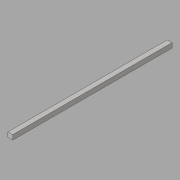
# Autodesk Inventor part: c1e
Saved by Autodesk Inventor 2016 (Build 200138000, 138)
## iProperties
Created: 2015-10-11
Part Number: c1e
Material: Generic
Document SubType Name: Modeling
Designer: daniel
Density: 1 g/cm^3
Appearance: Default
Author: daniel
Autodesk Inventor part; units mm, degrees
ref_plane "YZ Plane" through (0, 0, 0) normal (1, 0, 0) x (0, 1, 0)
ref_plane "XZ Plane" through (0, 0, 0) normal (0, 1, 0) x (-1, 0, 0)
ref_plane "XY Plane" through (0, 0, 0) normal (0, 0, 1) x (1, 0, 0)
derived "base.ipt"
sketch "sketch_projected_dwg" plane through (0, 0, 0) normal (0, 0, 1) x (1, 0, 0)
  line L0 (2002.0921, -140.1606) -> (2002.0921, -170.1606)
  line L1 (2002.0921, -170.1606) -> (2026.0921, -170.1606)
  line L2 (2026.0921, -170.1606) -> (2026.0921, -140.1606)
  line L3 (2026.0921, -140.1606) -> (2029.0921, -140.1606)
  line L4 (2029.0921, -140.1606) -> (2029.0921, -173.1606)
  line L5 (2029.0921, -173.1606) -> (2049.0921, -173.1606)
  line L6 (2049.0921, -173.1606) -> (2049.0921, -170.1606)
  line L7 (2049.0921, -170.1606) -> (2064.0921, -170.1606)
  line L8 (2064.0921, -170.1606) -> (2064.0921, -110.1606)
  line L9 (2064.0921, -110.1606) -> (2049.0921, -110.1606)
  line L10 (2049.0921, -110.1606) -> (2049.0921, -107.1606)
  line L11 (2049.0921, -107.1606) -> (2029.0921, -107.1606)
  line L12 (2029.0921, -107.1606) -> (2029.0921, -110.1606)
  line L13 (2029.0921, -110.1606) -> (1999.0921, -110.1606)
  line L14 (1999.0921, -110.1606) -> (1999.0921, -107.1606)
  line L15 (1999.0921, -107.1606) -> (1979.0921, -107.1606)
  line L16 (1979.0921, -107.1606) -> (1979.0921, -110.1606)
  line L17 (1979.0921, -110.1606) -> (1964.0921, -110.1606)
  line L18 (1964.0921, -110.1606) -> (1964.0921, -170.1606)
  line L19 (1964.0921, -170.1606) -> (1979.0921, -170.1606)
  line L20 (1979.0921, -170.1606) -> (1979.0921, -173.1606)
  line L21 (1979.0921, -173.1606) -> (1999.0921, -173.1606)
  line L22 (1999.0921, -173.1606) -> (1999.0921, -140.1606)
  line L23 (1999.0921, -140.1606) -> (2002.0921, -140.1606)
  line L24 (2002.0921, -228.8911) -> (2002.0921, -258.8911)
  line L25 (2002.0921, -258.8911) -> (1999.0921, -258.8911)
  line L26 (1999.0921, -258.8911) -> (1999.0921, -228.8911)
  line L27 (1999.0921, -228.8911) -> (1971.0921, -228.8911)
  line L28 (1971.0921, -228.8911) -> (1971.0921, -288.8911)
  line L29 (1971.0921, -288.8911) -> (2057.0921, -288.8911)
  line L30 (2057.0921, -288.8911) -> (2057.0921, -228.8911)
  line L31 (2057.0921, -228.8911) -> (2029.0921, -228.8911)
  line L32 (2029.0921, -228.8911) -> (2029.0921, -258.8911)
  line L33 (2029.0921, -258.8911) -> (2026.0921, -258.8911)
  line L34 (2026.0921, -258.8911) -> (2026.0921, -228.8911)
  line L35 (2026.0921, -228.8911) -> (2002.0921, -228.8911)
  circle A0 centre (2044.0921, -265.8911) radius 6
  circle A1 centre (2014.0921, -265.8911) radius 4.7571
  circle A2 centre (1984.0921, -265.8911) radius 6
  line L36 (2368.3683, 1.7867) -> (2368.3683, -98.2133)
  line L37 (2472.3683, 1.7867) -> (2472.3683, -98.2133)
  line L38 (2377.3683, -263.5692) -> (2377.3683, -363.5692)
  line L39 (2463.3683, -263.5692) -> (2463.3683, -363.5692)
  line L40 (2317.3683, -263.5692) -> (2377.3683, -263.5692)
  line L41 (2377.3683, -263.5692) -> (2420.3683, -263.5692)
  line L42 (2420.3683, -263.5692) -> (2463.3683, -263.5692)
  line L43 (2463.3683, -263.5692) -> (2523.3683, -263.5692)
  line L44 (2523.3683, -263.5692) -> (2523.3683, -333.5692)
  line L45 (2523.3683, -333.5692) -> (2493.3683, -363.5692)
  line L46 (2493.3683, -363.5692) -> (2347.3683, -363.5692)
  line L47 (2347.3683, -363.5692) -> (2317.3683, -333.5692)
  line L48 (2317.3683, -333.5692) -> (2317.3683, -263.5692)
  line L49 (2405.3683, -278.5692) -> (2408.3683, -278.5692)
  line L50 (2408.3683, -278.5692) -> (2408.3683, -298.5692)
  line L51 (2408.3683, -298.5692) -> (2405.3683, -298.5692)
  line L52 (2405.3683, -298.5692) -> (2405.3683, -278.5692)
  line L53 (2432.3683, -278.5692) -> (2435.3683, -278.5692)
  line L54 (2435.3683, -278.5692) -> (2435.3683, -298.5692)
  line L55 (2435.3683, -298.5692) -> (2432.3683, -298.5692)
  line L56 (2432.3683, -298.5692) -> (2432.3683, -278.5692)
  line L57 (2432.3683, -328.5692) -> (2435.3683, -328.5692)
  line L58 (2435.3683, -328.5692) -> (2435.3683, -348.5692)
  line L59 (2435.3683, -348.5692) -> (2432.3683, -348.5692)
  line L60 (2432.3683, -348.5692) -> (2432.3683, -328.5692)
  line L61 (2405.3683, -328.5692) -> (2408.3683, -328.5692)
  line L62 (2408.3683, -328.5692) -> (2408.3683, -348.5692)
  line L63 (2408.3683, -348.5692) -> (2405.3683, -348.5692)
  line L64 (2405.3683, -348.5692) -> (2405.3683, -328.5692)
  line L65 (2405.3683, -63.2133) -> (2408.3683, -63.2133)
  line L66 (2408.3683, -63.2133) -> (2408.3683, -83.2133)
  line L67 (2408.3683, -83.2133) -> (2405.3683, -83.2133)
  line L68 (2405.3683, -83.2133) -> (2405.3683, -63.2133)
  line L69 (2371.3683, -63.2133) -> (2374.3683, -63.2133)
  line L70 (2374.3683, -63.2133) -> (2374.3683, -83.2133)
  line L71 (2374.3683, -83.2133) -> (2371.3683, -83.2133)
  line L72 (2371.3683, -83.2133) -> (2371.3683, -63.2133)
  line L73 (2371.3683, -13.2133) -> (2374.3683, -13.2133)
  line L74 (2374.3683, -13.2133) -> (2374.3683, -33.2133)
  line L75 (2374.3683, -33.2133) -> (2371.3683, -33.2133)
  line L76 (2371.3683, -33.2133) -> (2371.3683, -13.2133)
  line L77 (2405.3683, -13.2133) -> (2408.3683, -13.2133)
  line L78 (2408.3683, -13.2133) -> (2408.3683, -33.2133)
  line L79 (2408.3683, -33.2133) -> (2405.3683, -33.2133)
  line L80 (2405.3683, -33.2133) -> (2405.3683, -13.2133)
  line L81 (2432.3683, -13.2133) -> (2435.3683, -13.2133)
  line L82 (2435.3683, -13.2133) -> (2435.3683, -33.2133)
  line L83 (2435.3683, -33.2133) -> (2432.3683, -33.2133)
  line L84 (2432.3683, -33.2133) -> (2432.3683, -13.2133)
  line L85 (2466.3683, -13.2133) -> (2469.3683, -13.2133)
  line L86 (2469.3683, -13.2133) -> (2469.3683, -33.2133)
  line L87 (2469.3683, -33.2133) -> (2466.3683, -33.2133)
  line L88 (2466.3683, -33.2133) -> (2466.3683, -13.2133)
  line L89 (2466.3683, -63.2133) -> (2469.3683, -63.2133)
  line L90 (2469.3683, -63.2133) -> (2469.3683, -83.2133)
  line L91 (2469.3683, -83.2133) -> (2466.3683, -83.2133)
  line L92 (2466.3683, -83.2133) -> (2466.3683, -63.2133)
  line L93 (2432.3683, -63.2133) -> (2435.3683, -63.2133)
  line L94 (2435.3683, -63.2133) -> (2435.3683, -83.2133)
  line L95 (2435.3683, -83.2133) -> (2432.3683, -83.2133)
  line L96 (2432.3683, -83.2133) -> (2432.3683, -63.2133)
  line L97 (2519.3683, -98.2133) -> (2469.3683, -98.2133)
  line L98 (2469.3683, 61.7867) -> (2519.3683, 61.7867)
  line L99 (2519.3683, 61.7867) -> (2519.3683, 1.7867)
  line L100 (2519.3683, 1.7867) -> (2595.3683, 1.7867)
  line L101 (2595.3683, 1.7867) -> (2595.3683, -13.2133)
  line L102 (2595.3683, -13.2133) -> (2598.3683, -13.2133)
  line L103 (2598.3683, -13.2133) -> (2598.3683, -33.2133)
  line L104 (2598.3683, -33.2133) -> (2595.3683, -33.2133)
  line L105 (2595.3683, -33.2133) -> (2595.3683, -48.2133)
  line L106 (2595.3683, -48.2133) -> (2595.3683, -63.2133)
  line L107 (2595.3683, -63.2133) -> (2598.3683, -63.2133)
  line L108 (2598.3683, -63.2133) -> (2598.3683, -83.2133)
  line L109 (2598.3683, -83.2133) -> (2595.3683, -83.2133)
  line L110 (2595.3683, -83.2133) -> (2595.3683, -98.2133)
  line L111 (2595.3683, -98.2133) -> (2519.3683, -98.2133)
  line L112 (2519.3683, -98.2133) -> (2519.3683, -158.2133)
  line L113 (2519.3683, -158.2133) -> (2394.6842, -158.2133)
  line L114 (2532.3683, 1.7867) -> (2532.3683, -98.2133)
  line L115 (2535.3683, 1.7867) -> (2535.3683, -98.2133)
  line L116 (2371.3683, -158.2133) -> (2371.3683, -98.2133)
  line L117 (2371.3683, -98.2133) -> (2469.3683, -98.2133)
  line L118 (2469.3683, -98.2133) -> (2469.3683, -158.2133)
  circle A3 centre (2450.3683, -121.2133) radius 6
  circle A4 centre (2428.6172, -116.4508) radius 1.5
  circle A5 centre (2420.3683, -121.2133) radius 6.35
  circle A6 centre (2412.1194, -116.4508) radius 1.5
  circle A7 centre (2420.3683, -130.7383) radius 1.5
  circle A8 centre (2390.3683, -121.2133) radius 6
  line L119 (2371.3683, -158.2133) -> (2420.3683, -158.2133)
  line L120 (2420.3683, -158.2133) -> (2469.3683, -158.2133)
  line L121 (2394.6842, -158.2133) -> (2321.3683, -158.2133)
  line L122 (2321.3683, -158.2133) -> (2321.3683, -98.2133)
  line L123 (2321.3683, -98.2133) -> (2245.3683, -98.2133)
  line L124 (2245.3683, -98.2133) -> (2245.3683, -83.2133)
  line L125 (2245.3683, -83.2133) -> (2242.3683, -83.2133)
  line L126 (2242.3683, -83.2133) -> (2242.3683, -63.2133)
  line L127 (2242.3683, -63.2133) -> (2245.3683, -63.2133)
  line L128 (2245.3683, -63.2133) -> (2245.3683, -48.2133)
  line L129 (2245.3683, -48.2133) -> (2245.3683, -33.2133)
  line L130 (2245.3683, -33.2133) -> (2242.3683, -33.2133)
  line L131 (2242.3683, -33.2133) -> (2242.3683, -13.2133)
  line L132 (2242.3683, -13.2133) -> (2245.3683, -13.2133)
  line L133 (2245.3683, -13.2133) -> (2245.3683, 1.7867)
  line L134 (2245.3683, 1.7867) -> (2321.3683, 1.7867)
  line L135 (2321.3683, 1.7867) -> (2321.3683, 61.7867)
  line L136 (2321.3683, -98.2133) -> (2371.3683, -98.2133)
  line L137 (2308.3683, 1.7867) -> (2308.3683, -98.2133)
  line L138 (2305.3683, 1.7867) -> (2305.3683, -98.2133)
  line L139 (2321.3683, 61.7867) -> (2371.3683, 61.7867)
  line L140 (2371.3683, 61.7867) -> (2420.3683, 61.7867)
  line L141 (2420.3683, 61.7867) -> (2469.3683, 61.7867)
  line L142 (2371.3683, 61.7867) -> (2371.3683, 1.7867)
  line L143 (2371.3683, 1.7867) -> (2469.3683, 1.7867)
  line L144 (2469.3683, 1.7867) -> (2469.3683, 61.7867)
  circle A9 centre (2390.3683, 24.7867) radius 6
  circle A10 centre (2420.3683, 24.7867) radius 4.5
  circle A11 centre (2450.3683, 24.7867) radius 6
  line L145 (2519.3683, 1.7867) -> (2469.3683, 1.7867)
  line L146 (2321.3683, 1.7867) -> (2371.3683, 1.7867)
  line L147 (1481.5912, 324.5306) -> (1293.5912, 324.5306)
  line L148 (1293.5912, 324.5306) -> (1293.5912, 259.5306)
  line L149 (1293.5912, 259.5306) -> (1481.5912, 259.5306)
  line L150 (1481.5912, 259.5306) -> (1599.5912, 259.5306)
  line L151 (1599.5912, 259.5306) -> (1787.5912, 259.5306)
  line L152 (1787.5912, 259.5306) -> (1787.5912, 324.5306)
  line L153 (1787.5912, 324.5306) -> (1599.5912, 324.5306)
  line L154 (1599.5912, 324.5306) -> (1481.5912, 324.5306)
  line L155 (1599.5912, 324.5306) -> (1599.5912, 259.5306)
  circle A12 centre (1570.5912, 294.5306) radius 5
  circle A13 centre (1556.0912, 310.0306) radius 1.5
  circle A14 centre (1556.0912, 279.0306) radius 1.5
  circle A15 centre (1540.5912, 294.5306) radius 4.5
  circle A16 centre (1510.5912, 294.5306) radius 5
  circle A17 centre (1525.0912, 279.0306) radius 1.5
  circle A18 centre (1525.0912, 310.0306) radius 1.5
  line L156 (1481.5912, 324.5306) -> (1481.5912, 259.5306)
  line L157 (1481.5912, 203.0466) -> (1481.5912, 138.0466)
  line L158 (1481.5912, 203.0466) -> (1293.5912, 203.0466)
  line L159 (1293.5912, 203.0466) -> (1293.5912, 138.0466)
  line L160 (1293.5912, 138.0466) -> (1787.5912, 138.0466)
  line L161 (1787.5912, 138.0466) -> (1787.5912, 203.0466)
  line L162 (1787.5912, 203.0466) -> (1599.5912, 203.0466)
  line L163 (1599.5912, 203.0466) -> (1481.5912, 203.0466)
  line L164 (1599.5912, 203.0466) -> (1599.5912, 138.0466)
  circle A19 centre (1570.5912, 173.0466) radius 5
  circle A20 centre (1540.5912, 173.0466) radius 4.5
  circle A21 centre (1510.5912, 173.0466) radius 5
  line L165 (1565.5912, 43.4562) -> (1515.5912, 43.4562)
  line L166 (1515.5912, 43.4562) -> (1515.5912, 37.4562)
  line L167 (1515.5912, 37.4562) -> (1515.5912, 18.4562)
  line L168 (1515.5912, 18.4562) -> (1565.5912, 18.4562)
  line L169 (1565.5912, 18.4562) -> (1565.5912, 37.4562)
  line L170 (1565.5912, 37.4562) -> (1565.5912, 43.4562)
  line L171 (1481.5912, 40.4562) -> (1515.5912, 40.4562)
  line L172 (1456.5912, 105.4562) -> (1456.5912, 40.4562)
  line L173 (1456.5912, 40.4562) -> (1481.5912, 40.4562)
  line L174 (1481.5912, 105.4562) -> (1481.5912, 40.4562)
  line L175 (1456.5912, 105.4562) -> (1481.5912, 105.4562)
  line L176 (1481.5912, 105.4562) -> (1599.5912, 105.4562)
  circle A22 centre (1510.5912, 75.4562) radius 5
  circle A23 centre (1540.5912, 75.4562) radius 4.5
  circle A24 centre (1570.5912, 75.4562) radius 5
  line L177 (1599.5912, 105.4562) -> (1599.5912, 40.4562)
  line L178 (1599.5912, 40.4562) -> (1565.5912, 40.4562)
  line L179 (1599.5912, 40.4562) -> (1624.5912, 40.4562)
  line L180 (1624.5912, 105.4562) -> (1624.5912, 40.4562)
  line L181 (1599.5912, 105.4562) -> (1624.5912, 105.4562)
  line L182 (1481.5912, -237.3994) -> (1599.5912, -237.3994)
  line L183 (1481.5912, -237.3994) -> (1481.5912, -302.3994)
  circle A25 centre (1525.0912, -251.8994) radius 1.5
  line L184 (1599.5912, -237.3994) -> (1599.5912, -302.3994)
  circle A26 centre (1570.5912, -267.3994) radius 5
  circle A27 centre (1556.0912, -251.8994) radius 1.5
  circle A28 centre (1556.0912, -282.8994) radius 1.5
  circle A29 centre (1525.0912, -282.8994) radius 1.5
  circle A30 centre (1540.5912, -267.3994) radius 11
  circle A31 centre (1510.5912, -267.3994) radius 5
  line L185 (1481.5912, -302.3994) -> (1515.5912, -302.3994)
  line L186 (1515.5912, -299.3994) -> (1515.5912, -305.3994)
  line L187 (1515.5912, -305.3994) -> (1515.5912, -324.3994)
  line L188 (1515.5912, -324.3994) -> (1565.5912, -324.3994)
  line L189 (1565.5912, -324.3994) -> (1565.5912, -305.3994)
  line L190 (1565.5912, -305.3994) -> (1565.5912, -299.3994)
  line L191 (1565.5912, -299.3994) -> (1515.5912, -299.3994)
  line L192 (1599.5912, -302.3994) -> (1565.5912, -302.3994)
  line L193 (618.8683, 258.8909) -> (618.8683, 505.8909)
  line L194 (618.8683, 505.8909) -> (553.8683, 505.8909)
  line L195 (553.8683, 505.8909) -> (553.8683, 332.8909)
  line L196 (553.8683, 332.8909) -> (550.8683, 332.8909)
  line L197 (550.8683, 332.8909) -> (550.8683, 417.8909)
  line L198 (550.8683, 417.8909) -> (500.8683, 417.8909)
  line L199 (500.8683, 417.8909) -> (500.8683, 332.8909)
  line L200 (500.8683, 332.8909) -> (494.8683, 332.8909)
  line L201 (494.8683, 332.8909) -> (494.8683, 437.8909)
  line L202 (494.8683, 437.8909) -> (118.8683, 437.8909)
  line L203 (118.8683, 437.8909) -> (118.8683, 332.8909)
  line L204 (118.8683, 332.8909) -> (112.8683, 332.8909)
  line L205 (112.8683, 332.8909) -> (112.8683, 417.8909)
  line L206 (112.8683, 417.8909) -> (62.8683, 417.8909)
  line L207 (62.8683, 417.8909) -> (62.8683, 332.8909)
  line L208 (62.8683, 332.8909) -> (59.8683, 332.8909)
  line L209 (59.8683, 332.8909) -> (59.8683, 505.8909)
  line L210 (59.8683, 505.8909) -> (-5.1317, 505.8909)
  line L211 (-5.1317, 505.8909) -> (-5.1317, 258.8909)
  line L212 (500.8683, 397.8909) -> (550.8683, 397.8909)
  line L213 (500.8683, 394.8909) -> (550.8683, 394.8909)
  line L214 (118.8683, 394.8909) -> (494.8683, 394.8909)
  line L215 (494.8683, 397.8909) -> (118.8683, 397.8909)
  line L216 (550.8683, 332.8909) -> (500.8683, 332.8909)
  line L217 (494.8683, 332.8909) -> (118.8683, 332.8909)
  line L218 (553.8683, 326.8909) -> (59.8683, 326.8909)
  line L219 (553.8683, 332.8909) -> (553.8683, 326.8909)
  line L220 (553.8683, 326.8909) -> (553.8683, 261.8909)
  line L221 (618.8683, 258.8909) -> (553.8683, 258.8909)
  line L222 (553.8683, 134.8909) -> (553.8683, 258.8909)
  line L223 (59.8683, 261.8909) -> (553.8683, 261.8909)
  line L224 (553.8683, 258.8909) -> (553.8683, 261.8909)
  line L225 (618.8683, 258.8909) -> (618.8683, 134.8909)
  circle A32 centre (588.8683, 226.8909) radius 5
  circle A33 centre (588.8683, 166.8909) radius 5
  line L226 (618.8683, 134.8909) -> (553.8683, 134.8909)
  line L227 (59.8683, 131.8909) -> (553.8683, 131.8909)
  line L228 (553.8683, 134.8909) -> (553.8683, 131.8909)
  line L229 (59.8683, 258.8909) -> (59.8683, 134.8909)
  line L230 (59.8683, 134.8909) -> (-5.1317, 134.8909)
  line L231 (59.8683, 134.8909) -> (59.8683, 131.8909)
  line L232 (59.8683, 258.8909) -> (59.8683, 261.8909)
  line L233 (-5.1317, 258.8909) -> (59.8683, 258.8909)
  line L234 (-5.1317, 258.8909) -> (-5.1317, 134.8909)
  circle A34 centre (24.8683, 226.8909) radius 5
  circle A35 centre (24.8683, 166.8909) radius 5
  line L235 (59.8683, 332.8909) -> (59.8683, 320.8909)
  line L236 (59.8683, 320.8909) -> (59.8683, 261.8909)
  line L237 (62.8683, 332.8909) -> (112.8683, 332.8909)
  line L238 (112.8683, 394.8909) -> (62.8683, 394.8909)
  line L239 (112.8683, 397.8909) -> (62.8683, 397.8909)
  line L240 (118.8683, 206.8909) -> (494.8683, 206.8909)
  line L241 (118.8683, 206.8909) -> (118.8683, 186.8909)
  line L242 (118.8683, 186.8909) -> (494.8683, 186.8909)
  line L243 (494.8683, 196.8909) -> (494.8683, 186.8909)
  line L244 (494.8683, 206.8909) -> (494.8683, 196.8909)
  point P0 (0, 0)
extrude "Extrusion1" add sketch "sketch_projected_dwg" along normal blind 3 contours L137 L123 L138 L134
equation "\"d1\" = material_thickness"
equation "\"material_thickness\" = 3"
body "Solid1"
